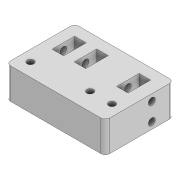
# Autodesk Inventor part: Bar_connection_block
Saved by Autodesk Inventor 2022 (Build 260153000, 153)
## iProperties
Created: 2022-08-24
Part Number: Bar_connection_block
Material: Generic
Document SubType Name: Modeling
Designer: dell
Density: 1 g/cm^3
Appearance: Default
Mass: 13.2571 g
Surface Area: 54.305 cm^2
Volume: 13.2571 cm^3
Author: dell
Autodesk Inventor part; units mm, degrees
ref_plane "YZ Plane" through (0, 0, 0) normal (1, 0, 0) x (0, 1, 0)
ref_plane "XZ Plane" through (0, 0, 0) normal (0, 1, 0) x (-1, 0, 0)
ref_plane "XY Plane" through (0, 0, 0) normal (0, 0, 1) x (1, 0, 0)
sketch "Sketch1" plane through (0, 0, 0) normal (0, 1, 0) x (-1, 0, 0)
  circle A0 centre (0, 0) radius 1.5
  circle A1 centre (25, 2) radius 1.5
  line L0 (30, 8) -> (-14.9, 8)
  line L1 (-14.9, 8) -> (-14.9, -23)
  line L2 (-14.9, -23) -> (30, -23)
  line L3 (30, -23) -> (30, 8)
  line L4 (-14.9, -8) -> (30, -8) construction
  circle A2 centre (-9.9, 0) radius 1.5
  line L5 (25, -8) -> (20, -8)
  line L6 (20, -8) -> (20, -18)
  line L7 (20, -18) -> (25, -18)
  line L8 (25, -18) -> (25, -8)
  line L9 (20, -8) -> (20, -18)
  line L10 (20, -18) -> (15, -18)
  line L11 (15, -18) -> (15, -8)
  line L12 (15, -8) -> (20, -8)
  line L13 (15, -8) -> (15, -18)
  line L14 (15, -18) -> (10, -18)
  line L15 (10, -18) -> (10, -8)
  line L16 (10, -8) -> (15, -8)
  line L17 (-4.2, -23) -> (-14.9, -23)
  line L18 (-14.9, -23) -> (-14.9, -8)
  line L19 (-9.2, -8) -> (-9.2, -18)
  line L20 (-9.2, -18) -> (-4.2, -18)
  line L21 (-4.2, -18) -> (-4.2, -8)
  line L22 (-4.2, -8) -> (-9.2, -8)
  dimension "d0" = 3
  dimension "d1" = 3
  dimension "d3" = 25
  dimension "d4" = 2
  dimension "d5" = 8
  dimension "d6" = 6
  dimension "d7" = 5
  dimension "d9" = 3
  dimension "d10" = 9.9
  dimension "d11" = 5
  dimension "d12" = 10
  dimension "d13" = 5
  dimension "d14" = 5
  dimension "d15" = 5
  dimension "d16" = 5
  dimension "d37" = 5
  dimension "d38" = 14.2
  dimension "d39" = 5
  constraints: 46 end point, 12 equal length, 8 perpendicular, 6 point on line, 3 centre point, 3 horizontal, 1 coincident, 1 horizontal alignment
  measures "d0" diameter of A0
  measures "d1" diameter of A1
  measures "d3" horizontal distance of point (0, 0) A1.centre
  measures "d4" vertical distance of point (0, 0) A1.centre
  measures "d5" distance from line of point (0, 0) L4
  measures "d6" distance from line of L0 A1.centre
  measures "d7" distance from line of A1.centre L3
  measures "d9" diameter of A2
  measures "d10" distance of point (0, 0) A2.centre
  measures "d11" distance from line of L1 A2.centre
  measures "d12" distance of L5.end L6.end
  measures "d13" distance of L6.end L7.end
  measures "d14" distance of L6.end L10.end
  measures "d15" distance of L10.end L14.end
  measures "d16" distance between parallel lines of L7 L2
  measures "d37" distance between parallel lines of L19 L21
  measures "d38" distance between parallel lines of L15 L21
  measures "d39" distance between parallel lines of L2 L20
extrude "Extrusion1" add sketch "Sketch1" along normal blind 14 contours L3 L2 L1 L0 | L6 L10 L11 L12
fillet "Fillet1" radius 2 4 edges at (-30, 7, 8) (-30, 7, -23) (14.9, 7, 8) (14.9, 7, -23)
sketch "Sketch2" plane through (-30, 0, -21) normal (-1, 0, 0) x (0, 0, 1)
  line L0 (3, 0) -> (13, 0) projected
  line L1 (13, 0) -> (13, 14) projected
  line L2 (3, 14) -> (13, 14) projected
  line L3 (3, 0) -> (3, 14) projected
  circle A0 centre (8, 11) radius 1.55
  circle A1 centre (8, 3) radius 1.55
  line L4 (3, 0) -> (3, 14) projected
  point P0 (21, 0)
  dimension "d21" = 3.1
  dimension "d22" = 3.1
  dimension "d23" = 3
  dimension "d24" = 3
  dimension "d35" = 5
  dimension "d36" = 5
  constraints: 2 centre point
  measures "d21" diameter of A0
  measures "d22" diameter of A1
  measures "d23" distance from line of L2 A0.centre
  measures "d24" distance from line of L0 A1.centre
  measures "d35" distance from line of L4 A0.centre
  measures "d36" distance from line of L3 A1.centre
extrude "Extrusion2" cut sketch "Sketch2" against normal blind 50 contours A0 | A1
thicken "Thicken1" operation add thickness 0.1 both sides no extend neighbours yes toward (1, 0, 0) faces at (-20, 8.0932, -9.2092) (-21.6667, 4.6667, -8) (-25, 8.0932, -9.2092) (-23.3333, 4.6667, -18)
thicken "Thicken2" operation add thickness 0.1 both sides no extend neighbours yes toward (0, 0, 1) faces at (-11.6667, 4.6667, -8) (-15, 8.0932, -9.2092) (-13.3333, 4.6667, -18) (-10, 5.9068, -16.7908)
thicken "Thicken3" operation add thickness 0.1 both sides no extend neighbours yes toward (-1, 0, 0) faces at (4.2, 8.0932, -16.7908) (5.8667, 4.6667, -18) (9.2, 5.9068, -16.7908) (7.5333, 4.6667, -8)
body "Solid1"
